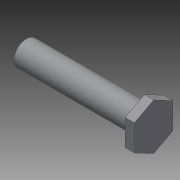
# Autodesk Inventor part: 8mm_x_rail_connection
Saved by Autodesk Inventor 2015 (Build 190159000, 159)
## iProperties
Created: 2017-03-25
Part Number: 8mm_x_rail_connection
Material: Generic
Document SubType Name: Modeling
Designer: Guy
Density: 1 g/cm^3
Appearance: Default
Mass: 2.35119 g
Surface Area: 13.8309 cm^2
Volume: 2.35119 cm^3
Author: Guy
Autodesk Inventor part; units mm, degrees
ref_plane "YZ Plane" through (0, 0, 0) normal (1, 0, 0) x (0, 1, 0)
ref_plane "XZ Plane" through (0, 0, 0) normal (0, 1, 0) x (-1, 0, 0)
ref_plane "XY Plane" through (0, 0, 0) normal (0, 0, 1) x (1, 0, 0)
sketch "Sketch1" plane through (0, 0, 0) normal (0, 0, 1) x (1, 0, 0)
  line L0 (0, 0) -> (0, 4)
  line L1 (0, 4) -> (38.1, 4)
  line L2 (38.1, 4) -> (38.1, 7.5)
  line L3 (38.1, 7.5) -> (41.1, 7.5)
  line L4 (41.1, 7.5) -> (41.1, 0)
  line L5 (41.1, 0) -> (0, 0)
  dimension "d0" = 4
  dimension "d1" = 38.1
  dimension "d2" = 3
  dimension "d3" = 7.5
  constraints: 12 end point, 5 perpendicular, 1 vertical
  measures "d0" distance between parallel lines of L5 L1
  measures "d1" distance of L0.end L1.end
  measures "d2" distance of L2.end L3.end
  measures "d3" distance between parallel lines of L5 L3
revolve "Revolution1" add sketch "Sketch1" angle 360 about axis through (41.1, 0, 0) along (-1, 0, 0)
sketch "Sketch2" plane through (41.1, 0, 0) normal (1, 0, 0) x (0, 0, -1)
  circle A0 centre (0, 0) radius 7.5 projected
  line L0 (-4.212, 6.2056) -> (4.212, 6.2056)
  line L1 (7.5, 0) -> (4.212, 6.2056)
  line L2 (7.5, 0) -> (4.212, -6.2056)
  line L3 (4.212, -6.2056) -> (-4.212, -6.2056)
  line L4 (-4.212, -6.2056) -> (-7.5, 0)
  line L5 (-4.212, 6.2056) -> (-7.5, 0)
  constraints: 12 end point, 6 point on circle, 2 parallel, 1 horizontal
extrude "Extrusion1" cut sketch "Sketch2" against normal up to next contours L1 A0 | A0 L2 | L0 A0 | A0 L3 | L5 A0 | A0 L4
body "Solid1"
